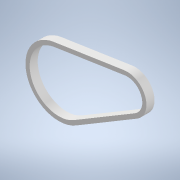
# Autodesk Inventor part: gumka1
Saved by Autodesk Inventor 2022.3 (Build 263350000, 350)
## iProperties
Created: 2022-12-14
Part Number: gumka1
Material: Generic
Document SubType Name: Modeling
Designer: komputer
Density: 1 g/cm^3
Appearance: Default
Author: komputer
Autodesk Inventor part; units mm, degrees
ref_plane "YZ Plane" through (0, 0, 0) normal (1, 0, 0) x (0, 1, 0)
ref_plane "XZ Plane" through (0, 0, 0) normal (0, 1, 0) x (-1, 0, 0)
sketch "Sketch1" plane through (0, 0, 0) normal (0, 0, 1) x (1, 0, 0)
  circle A0 centre (0, 0) radius 3.6028 projected
  line L0 (7.011, 4.2884) -> (7.2242, 4.5036) projected
  line L1 (8.945, 1.1673) -> (8.646, 1.1184) projected
  circle A1 centre (8.485, 3.042) radius 1 projected
  circle A2 centre (8.485, 3.042) radius 1.868
  circle A3 centre (0, 0) radius 4.1192
  circle A4 centre (8.485, 3.042) radius 2.3844
  line L2 (8.1274, 5.3994) -> (-0.6179, 4.0726)
  line L3 (2.1104, -3.5375) -> (9.7067, 0.9944)
  line L4 (-0.5404, 3.5621) -> (8.2048, 4.8889)
  line L5 (1.8459, -3.094) -> (9.4421, 1.4378)
  point P0 (0, 0)
  constraints: 8 end point, 8 point on circle, 8 tangent, 3 centre point, 3 coincident, 1 parallel
ref_plane "Work Plane1" through (-3.6028, -3.6028, 1) normal (0, 0, -1) x (0, 1, 0)
extrude "Extrusion1" add sketch "Sketch1" along normal up to surface (1 mm away) contours A0 L5 A3 L4 | A3 L2 A4 L4 | L5 A4 L3 A3 | A4 L5 A2 L4 picked at (2.8564, -2.6014) picked at (8.771, 0.9279)
chamfer "Chamfer1" distance 0.2 angle 45 8 edges at (3.8322, 4.2255, 1) (10.2435, 3.6725, 1) (5.644, -0.8281, 1) (-3.3914, -1.2159, 1) (3.8322, 4.2255, 0) (10.2435, 3.6725, 0) (5.644, -0.8281, 0) (-3.3914, -1.2159, 0)
body "Solid1"
